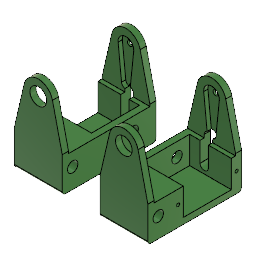
Leg_support (Autodesk Fusion 360 design; units mm, degrees)
Autodesk Fusion 360 part; units mm, degrees
sketch "Sketch1" plane through (0, 0, 0) normal (0, 0, 1) x (1, 0, 0)
  line L0 (11.5, -22.5) -> (-11.5, -22.5)
  line L1 (-11.5, -22.5) -> (-11.5, 22.5)
  line L2 (-11.5, 22.5) -> (11.5, 22.5)
  line L3 (11.5, 22.5) -> (11.5, -22.5)
  line L4 (11.5, -22.5) -> (-11.5, 22.5) construction
  line L5 (-11.5, -22.5) -> (11.5, 22.5) construction
  dimension "d1" = 45
  dimension "d2" = 23
  constraint perpendicular L0 L1
  constraint parallel L0 L2
  constraint parallel L1 L3
  constraint horizontal L0
  constraint coincident L4 origin
  constraint coincident L5 origin
  measures "d1" distance of L0.end L1.end
  measures "d2" distance of L1.end L2.end
extrude "Extrude1" add sketch "Sketch1" along normal blind 3 makes body 1
sketch "Sketch2" plane through (0, 0, 3) normal (0, 0, 1) x (-1, 0, 0)
  line L0 (-11.5, -22.5) -> (11.5, -22.5)
  line L1 (11.5, -22.5) -> (11.5, 22.5)
  line L2 (11.5, 22.5) -> (-11.5, 22.5)
  line L3 (-11.5, 22.5) -> (-11.5, -22.5)
  line L4 (11.5, -22.5) -> (-11.5, -22.5)
  line L5 (-11.5, -22.5) -> (-11.5, -19.5)
  line L6 (-11.5, -19.5) -> (11.5, -19.5)
  line L7 (11.5, -19.5) -> (11.5, -22.5)
  line L8 (11.5, 22.5) -> (-11.5, 22.5)
  line L9 (-11.5, 22.5) -> (-11.5, 19.5)
  line L10 (-11.5, 19.5) -> (11.5, 19.5)
  line L11 (11.5, 19.5) -> (11.5, 22.5)
  line L12 (11.5, -22.5) -> (-11.5, -22.5)
  line L13 (-11.5, -22.5) -> (-11.5, -17.5)
  line L14 (-11.5, -17.5) -> (11.5, -17.5)
  line L15 (11.5, -17.5) -> (11.5, -22.5)
  line L16 (11.5, 5.5) -> (-11.5, 5.5)
  line L17 (-11.5, 5.5) -> (-11.5, 10.5)
  line L18 (-11.5, 10.5) -> (11.5, 10.5)
  line L19 (11.5, 10.5) -> (11.5, 5.5)
  dimension "d5" = 3
  dimension "d6" = 3
  dimension "d9" = 5
  dimension "d10" = 5
  dimension "d11" = 23
  constraint horizontal L4
  constraint vertical L5
  constraint horizontal L6
  constraint vertical L7
  constraint coincident L0.end L1.start
  constraint horizontal L8
  constraint vertical L9
  constraint horizontal L10
  constraint vertical L11
  constraint coincident L1.end L2.start
  constraint horizontal L12
  constraint vertical L13
  constraint horizontal L14
  constraint vertical L15
  constraint horizontal L16
  constraint vertical L17
  constraint horizontal L18
  constraint vertical L19
  constraint coincident L1 L16.start
  constraint coincident L3 L5.end
  constraint coincident L3 L13.end
  constraint coincident L2.end L3.start
  measures "d5" distance of L0.end L6.end
  measures "d6" distance of L1.end L10.end
  measures "d9" distance of L0.end L14.end
  measures "d10" distance of L16.start L18.end
  measures "d11" distance of L13.end L16.end
extrude "Extrude5" add sketch "Sketch2" along normal blind 40 contours L0 L1 L3 L4 L5 L6 L7 L12 L13 L15 | L1 L2 L3 L8 L9 L10 L11 bodies 1
extrude "Extrude3" add sketch "Sketch2" along normal blind 13 contours L0 L1 L3 L4 L5 L6 L7 L12 L13 L15 | L1 L3 L6 L13 L14 L15 | L1 L3 L16 L17 L18 L19 | L1 L3 L10 L18 bodies 1
sketch "Sketch3" plane through (11.5, 0, 0) normal (1, 0, 0) x (0, 1, 0)
  line L0 (-22.5, 0) -> (22.5, 0)
  line L1 (22.5, 0) -> (22.5, 43)
  line L2 (-5.5, 16) -> (-19.5, 16)
  line L3 (17.5, 16) -> (17.5, 3)
  line L4 (17.5, 3) -> (-5.5, 3)
  line L5 (-5.5, 3) -> (-5.5, 16)
  line L6 (-22.5, 43) -> (-22.5, 0)
  line L7 (-6, 0) -> (-11, 0) construction
  line L8 (-19.5, 16) -> (-19.5, 43)
  line L9 (-19.5, 43) -> (-22.5, 43)
  line L10 (22.5, 43) -> (19.5, 43)
  line L11 (19.5, 43) -> (19.5, 16)
  line L12 (19.5, 16) -> (17.5, 16)
  circle A0 centre (11.5, 9.5) radius 2.5
  circle A1 centre (-17.5, 9.5) radius 2.5
  line L13 (-17.5, 9.5) -> (11.5, 9.5) construction
  line L14 (-5.5, 16) -> (17.5, 16) construction
  line L15 (11.5, 16) -> (11.5, 3) construction
  point P0 (-5.5, 3)
  dimension "d17" = 13
  dimension "d28" = 5
  dimension "d30" = 6
  dimension "d32" = 5
  dimension "d33" = 29
  constraint horizontal L7
  constraint coincident L0 L7.start
  constraint coincident A1.centre L13.start
  constraint coincident A0.centre L13.end
  constraint parallel L0 L13
  constraint coincident L2.start L5.end
  constraint coincident L3.start L12.end
  constraint coincident L14 L15.start
  constraint perpendicular L14 L15
  constraint coincident L4 L15.end
  constraint midpoint A0.centre L15
  measures "d17" distance of L2.start P0
  measures "d28" diameter of A0
  measures "d30" horizontal distance of L3.start A0.centre
  measures "d32" diameter of A1
  measures "d33" distance of A0.centre A1.centre
extrude "Extrude17" cut sketch "Sketch3" against normal through all contours A1 bodies 1
sketch "Sketch5" plane through (0, -19.5, 0) normal (0, 1, 0) x (-1, 0, 0)
  line L0 (-11.5, 16) -> (11.5, 16)
  line L1 (11.5, 16) -> (11.5, 43)
  line L2 (11.5, 43) -> (-11.5, 43)
  line L3 (-11.5, 43) -> (-11.5, 16)
  circle A0 centre (0, 35.5) radius 4
  dimension "d38" = 8
  dimension "d39" = 7.5
  measures "d38" diameter of A0
  measures "d39" distance of L2 A0.centre
extrude "Extrude8" cut sketch "Sketch5" against normal through all contours A0 bodies 1
sketch "Sketch6" plane through (0, 19.5, 0) normal (0, -1, 0) x (1, 0, 0)
  line L0 (-11.5, 16) -> (11.5, 16)
  line L1 (11.5, 16) -> (11.5, 43)
  line L2 (11.5, 43) -> (-11.5, 43)
  line L3 (-11.5, 43) -> (-11.5, 16)
  circle A0 centre (0, 35.5) radius 1.25
  circle A1 centre (0, 35.5) radius 3.75
  circle A2 centre (0, 19.5) radius 2.1
  line L4 (2.0888, 19.2834) -> (3.73, 35.1133)
  line L5 (-2.0888, 19.2834) -> (-3.73, 35.1133)
  line L6 (0, 68.2668) -> (0, 17.7332) construction
  dimension "d41" = 2.5
  dimension "d42" = 7.5
  dimension "d44" = 7.5
  dimension "d45" = 4.2
  dimension "d46" = 16
  constraint coincident A2 L4.start
  constraint coincident A2 L5.start
  constraint tangent A2 L5
  constraint tangent A2 L4
  constraint perpendicular L2 L6
  constraint midpoint L2 L6
  constraint coincident A2.centre L6
  constraint coincident A0.centre L6
  constraint coincident A1 L4.end
  constraint tangent A1 L4
  constraint coincident A1 L5.end
  constraint tangent A1 L5
  measures "d41" diameter of A0
  measures "d42" distance of L2 A0.centre
  measures "d44" diameter of A1
  measures "d45" diameter of A2
  measures "d46" distance of A0.centre A2.centre
extrude "Extrude10" cut sketch "Sketch6" against normal blind 2 contours A0 | A1 | A1 A2 L4 L5 | A2 bodies 1
extrude "Extrude11" cut sketch "Sketch6" against normal through all contours A0 bodies 1
chamfer "Chamfer1" distance 6 distance2 26 4 edges at (11.5, -21, 43) (11.5, 21, 43) (-11.5, 21, 43) (-11.5, -21, 43) measured on face at (-3.8333, -21.5, 43) measured on face at (3.8333, 20.5, 43) measured on face at (3.8333, 20.5, 43) measured on face at (-3.8333, -21.5, 43) on bodies 1
fillet "Fillet1" radius 7 4 edges at (5.5, -21, 43) (-5.5, -21, 43) (-5.5, 21, 43) (5.5, 21, 43) on bodies 1
fillet "Fillet2" radius 1.5 2 edges at (0, -22.5, 0) (0, 22.5, 0) on bodies 1
copy_body "CopyPasteBodies1" bodies 1 makes body 2
move_body "Move1" bodies 2 to x (1, 0, 0) y (0, 1, 0) z (0, 0, 1) at (-41, 0, 0)
sketch "Sketch4" plane through (0, 17.5, 0) normal (0, -1, 0) x (1, 0, 0)
  line L0 (-11.5, 3) -> (11.5, 3)
  line L1 (11.5, 3) -> (11.5, 16)
  line L2 (11.5, 16) -> (-11.5, 16)
  line L3 (-3.5, 17.5) -> (-3.5, 6.5)
  arc A0 (-3.5, 6.5) -> (0.5, 6.5) centre (-1.5, 6.5) ccw
  line L4 (0.5, 6.5) -> (0.5, 17.5)
  arc A1 (0.5, 17.5) -> (-3.5, 17.5) centre (-1.5, 17.5) ccw
  line L5 (-1.5, 17.5) -> (-1.5, 6.5) construction
  line L6 (-41.5, 17.5) -> (-41.5, 6.5)
  line L7 (-39.5, 17.5) -> (-39.5, 6.5) construction
  arc A2 (-41.5, 6.5) -> (-37.5, 6.5) centre (-39.5, 6.5) ccw
  line L8 (-37.5, 6.5) -> (-37.5, 17.5)
  arc A3 (-37.5, 17.5) -> (-41.5, 17.5) centre (-39.5, 17.5) ccw
  line L9 (-1.5, 12) -> (-39.5, 12) construction
  line L10 (11.5, 0) -> (-11.5, 0)
  line L11 (-52.5, 3) -> (-52.5, 16)
  line L12 (-29.5, 3) -> (-52.5, 3)
  point P0 (-1.5, 12)
  point P1 (11.5, 9.5)
  point P2 (-39.5, 12)
  point P3 (-37.5, 16)
  dimension "d34" = 5.5
  dimension "d35" = 4
  dimension "d57" = 13
  dimension "d58" = 5.5
  dimension "d59" = 4
  dimension "d79" = 13
  dimension "d95" = 3.5
  dimension "d96" = 3.5
  constraint tangent L3 A0
  constraint tangent A0 L4
  constraint parallel L3 L4
  constraint tangent L4 A1
  constraint tangent L3 A1
  constraint midpoint L5 P0
  constraint tangent L6 A2
  constraint tangent A2 L8
  constraint parallel L6 L8
  constraint tangent L8 A3
  constraint tangent L6 A3
  constraint midpoint P2 L7
  constraint parallel L5 L7
  constraint coincident P0 L9.start
  constraint coincident P2 L9.end
  constraint perpendicular L5 L9
  measures "d34" distance of A0.centre P0
  measures "d35" diameter of A0
  measures "d57" horizontal distance of P0 P1
  measures "d58" distance of L7.end P2
  measures "d59" diameter of A2
  measures "d79" distance of P2 L11
  measures "d95" distance of L7.end L12
  measures "d96" distance of L0 A0.centre
extrude "Extrude12" cut sketch "Sketch4" against normal through all bodies 1 2
sketch "Sketch7" plane through (11.5, 0, 0) normal (1, 0, 0) x (0, 1, 0)
  arc A0 (21, 0) -> (22.5, 1.5) centre (21, 1.5) ccw
  line L0 (22.5, 1.5) -> (22.5, 17)
  line L1 (22.5, 17) -> (19.5, 17)
  line L2 (17.5, 16) -> (17.5, 3)
  line L3 (17.5, 3) -> (-5.5, 3)
  line L4 (-5.5, 3) -> (-5.5, 16)
  line L5 (-19.5, 17) -> (-22.5, 17)
  line L6 (-22.5, 17) -> (-22.5, 1.5)
  arc A1 (-22.5, 1.5) -> (-21, 0) centre (-21, 1.5) ccw
  line L7 (-21, 0) -> (21, 0)
  circle A2 centre (-8, 9.5) radius 0.75
  line L8 (-8, 9.5) -> (20, 9.5) construction
  line L9 (-5.5, 3) -> (17.5, 16) construction
  circle A3 centre (20, 9.5) radius 0.75
  circle A4 centre (-17.5, 9.5) radius 2.5
  line L10 (19.5, 17) -> (19.5, 16)
  line L11 (19.5, 16) -> (17.5, 16)
  line L12 (-5.5, 16) -> (-19.5, 16)
  line L13 (-19.5, 16) -> (-19.5, 17)
  point P0 (17.5, 16)
  dimension "d64" = 1.5
  dimension "d69" = 1.5
  dimension "d94" = 28
  constraint coincident A2.centre L8.start
  constraint parallel L3 L8
  constraint coincident L3.end L4.start
  constraint midpoint L8 L9
  constraint coincident P0 L2.start
  measures "d64" diameter of A2
  measures "d69" diameter of A3
  measures "d94" distance of A2.centre L8.end
extrude "Extrude13" cut sketch "Sketch7" against normal blind 10 contours A2 | A3 bodies 1
sketch "Sketch8" plane through (-52.5, 0, 0) normal (-1, 0, 0) x (0, -1, 0)
  arc A0 (-22.5, 1.5) -> (-21, 0) centre (-21, 1.5) ccw
  line L0 (-21, 0) -> (21, 0)
  arc A1 (21, 0) -> (22.5, 1.5) centre (21, 1.5) ccw
  line L1 (22.5, 1.5) -> (22.5, 17)
  line L2 (22.5, 17) -> (19.5, 17)
  line L3 (-22.5, 17) -> (-22.5, 1.5)
  line L4 (5.5, 16) -> (5.5, 3)
  line L5 (5.5, 3) -> (-17.5, 3)
  line L6 (-17.5, 3) -> (-17.5, 16)
  circle A2 centre (8, 9.5) radius 0.75
  circle A3 centre (-20, 9.5) radius 0.75
  line L7 (-20, 9.5) -> (8, 9.5) construction
  line L8 (-17.5, 16) -> (5.5, 3) construction
  circle A4 centre (17.5, 9.5) radius 2.5
  line L9 (19.5, 17) -> (19.5, 16)
  line L10 (19.5, 16) -> (5.5, 16)
  line L11 (-17.5, 16) -> (-19.5, 16)
  line L12 (-19.5, 16) -> (-19.5, 17)
  line L13 (-19.5, 17) -> (-22.5, 17)
  dimension "d74" = 1.5
  dimension "d75" = 1.5
  dimension "d76" = 28
  constraint coincident A3.centre L7.start
  constraint coincident A2.centre L7.end
  constraint parallel L5 L7
  constraint coincident L6.end L8.start
  constraint coincident L4.end L5.start
  constraint midpoint L7 L8
  measures "d74" diameter of A2
  measures "d75" diameter of A3
  measures "d76" horizontal distance of A2.centre A3.centre
extrude "Extrude14" cut sketch "Sketch8" against normal blind 10 contours A2 | A3 bodies 2
sketch "Sketch11" plane through (0, 0, 3) normal (0, 0, 1) x (-1, 0, 0)
  line L0 (11.5, 5.5) -> (-11.5, 5.5)
  line L1 (-11.5, 5.5) -> (-11.5, -17.5)
  line L2 (-11.5, -17.5) -> (11.5, -17.5)
  line L3 (11.5, -17.5) -> (11.5, 5.5)
  line L4 (11.5, -17.5) -> (8.5, -17.5)
  line L5 (8.5, -17.5) -> (8.5, 5.5)
  line L6 (8.5, 5.5) -> (11.5, 5.5)
  line L7 (11.5, 5.5) -> (11.5, -17.5)
  dimension "d83" = 3
  constraint horizontal L4
  constraint vertical L5
  constraint horizontal L6
  constraint vertical L7
  constraint coincident L2.end L3.start
  measures "d83" distance of L2.end L4.end
extrude "Extrude15" add sketch "Sketch11" along normal blind 13 contours L0 L2 L3 L4 L5 L6 L7 bodies 1
sketch "Sketch12" plane through (0, 0, 3) normal (0, 0, 1) x (-1, 0, 0)
  line L0 (52.5, 5.5) -> (29.5, 5.5)
  line L1 (29.5, 5.5) -> (29.5, -17.5)
  line L2 (29.5, -17.5) -> (52.5, -17.5)
  line L3 (52.5, -17.5) -> (52.5, 5.5)
  line L4 (29.5, -17.5) -> (32.5, -17.5)
  line L5 (32.5, -17.5) -> (32.5, 5.5)
  line L6 (32.5, 5.5) -> (29.5, 5.5)
  line L7 (29.5, 5.5) -> (29.5, -17.5)
  dimension "d86" = 3
  constraint horizontal L4
  constraint vertical L5
  constraint horizontal L6
  constraint vertical L7
  constraint coincident L1.end L2.start
  measures "d86" distance of L1.end L4.end
extrude "Extrude16" add sketch "Sketch12" along normal blind 13 contours L0 L1 L2 L4 L5 L6 L7 bodies 2
extrude "Extrude19" cut sketch "Sketch3" against normal through all contours A0 bodies 1 2
named bodies: "Avant_Bras_1", "Avant_Bras_2"
